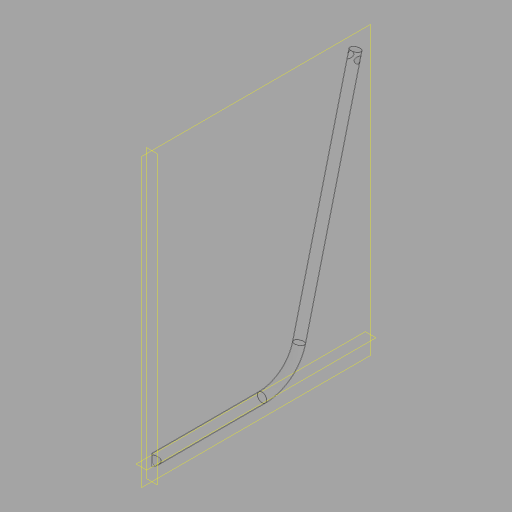
# Autodesk Inventor part: Hebel
Saved by Autodesk Inventor 2023.2 (Build 272271000, 271)
## iProperties
Created: 2023-02-02
Part Number: Hebel
Material: Generisch
Document SubType Name: Modeling
Designer: Raoul Messerli
Density: 1 g/cm^3
Appearance: Vorgabe
Author: Raoul Messerli
Autodesk Inventor part; units mm, degrees
sketch "Skizze2" plane through (0, 0, 0) normal (1, 0, 0) x (0, 1, 0)
  line L0 (0, 0) -> (865.7671, 0)
  arc A0 (865.7671, 0) -> (1156.8098, 227.2393) centre (865.7671, 300) ccw
  line L1 (1156.8098, 227.2393) -> (1600, 2000)
  line L2 (1156.8098, 227.2393) -> (1100, 0)
  line L3 (865.7671, 0) -> (1100, 0)
  dimension "d6" = 300
  dimension "d7" = 1600
  dimension "d8" = 2000
  dimension "d18" = 1100
  constraints: 8 end point, 3 tangent, 2 horizontal, 2 point on circle, 1 centre point, 1 coincident
  measures "d6" radius of A0
  measures "d7" horizontal distance of L0.start L1.end
  measures "d8" distance from line of L1.end L0
  measures "d18" distance of L0.start L2.end
sketch "Skizze3" plane through (0, 0, 0) normal (0, 1, 0) x (-1, 0, 0)
  circle A0 centre (0, 0) radius 38.05
  circle A1 centre (0, 0) radius 34.45
  dimension "d12" = 76.1
  dimension "d13" = 3.6
  constraints: 2 centre point, 2 coincident
  measures "d12" diameter of A0
  measures "d13" radial gap between concentric circles of A1 A0
sweep "Sweeping1" add profiles "Skizze3" path "Skizze2" path curves L0 A0 L1
sketch "Skizze5" plane through (0, 0, 0) normal (1, 0, 0) x (0, 1, 0)
  line L0 (0, -38.05) -> (0, 38.05) projected
  circle A0 centre (0, 0) radius 38.05
  constraints: 1 coincident, 1 vertical alignment, 2 other
extrude "Extrusion3" cut sketch "Skizze5" along normal mid plane 76.1
sketch "Skizze6" plane through (0, 0, 0) normal (1, 0, 0) x (0, 1, 0)
  line L0 (1636.9139, 1990.7715) -> (1563.0861, 2009.2285) projected
  line L1 (1600, 2000) -> (1587.8732, 1951.4929)
  circle A0 centre (1587.8732, 1951.4929) radius 25
  point P0 (0, 0)
  dimension "d19" = 50
  dimension "d21" = 50
  constraints: 2 end point, 1 centre point, 1 coincident, 1 midpoint, 1 perpendicular
  measures "d19" diameter of A0
  measures "d21" distance of L1.start L1.end
extrude "Extrusion4" cut sketch "Skizze6" along normal through all both and the other way through all
